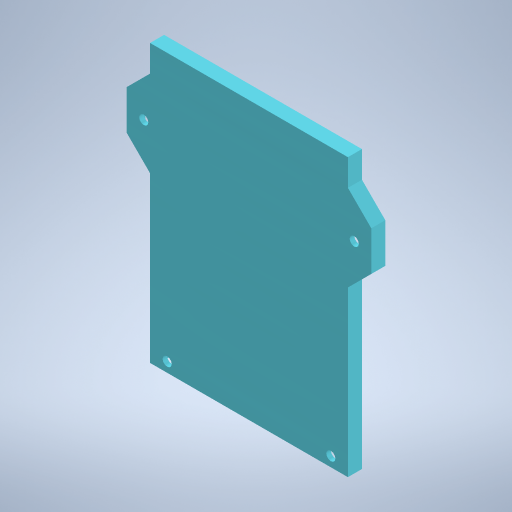
# Autodesk Inventor part: Cover
Saved by Autodesk Inventor 2024.2 (Build 282272000, 272)
## iProperties
Created: 2024-06-02
Part Number: Cover
Material: PBT Plastic
Document SubType Name: Modeling
Designer: simon
Density: 1.31 g/cm^3
Appearance: Cadet Blue
Author: simon
Autodesk Inventor part; units mm, degrees
ref_plane "YZ Plane" through (0, 0, 0) normal (1, 0, 0) x (0, 1, 0)
ref_plane "XZ Plane" through (0, 0, 0) normal (0, 1, 0) x (-1, 0, 0)
ref_plane "XY Plane" through (0, 0, 0) normal (0, 0, 1) x (1, 0, 0)
sketch "Sketch3" plane through (0, 0, 0) normal (0, 0, 1) x (1, 0, 0)
  line L0 (-10, 81) -> (0, 71) projected
  line L1 (-10, 96) -> (-10, 81) projected
  line L2 (0, 106) -> (-10, 96) projected
  line L3 (0, 116) -> (0, 106) projected
  line L4 (80, 116) -> (0, 116) projected
  line L5 (80, 106) -> (80, 116) projected
  line L6 (90, 96) -> (80, 106) projected
  line L7 (90, 81) -> (90, 96) projected
  line L8 (80, 71) -> (90, 81) projected
  line L9 (80, -0.1962) -> (80, 71) projected
  circle A0 centre (85, 88.5) radius 1.95 projected
  circle A1 centre (75, 4) radius 1.95 projected
  circle A2 centre (5, 4) radius 1.95 projected
  circle A3 centre (-5, 88.5) radius 1.95 projected
  line L10 (80, -0.1962) -> (80, 71)
  line L11 (80, 71) -> (90, 81)
  line L12 (90, 81) -> (90, 96)
  line L13 (90, 96) -> (80, 106)
  line L14 (80, 106) -> (80, 116)
  line L15 (80, 116) -> (0, 116)
  line L16 (0, 116) -> (0, 106)
  line L17 (0, 106) -> (-10, 96)
  line L18 (-10, 96) -> (-10, 81)
  line L19 (-10, 81) -> (0, 71)
  line L20 (80, -0.1962) -> (0, -0.1962)
  line L21 (0, 71) -> (0, -0.1962) projected
  line L22 (0, -0.1962) -> (0, 71)
  circle A4 centre (5, 4) radius 1.65
  circle A5 centre (-5, 88.5) radius 1.65
  circle A6 centre (85, 88.5) radius 1.65
  circle A7 centre (75, 4) radius 1.65
  line L23 (0, -0.1962) -> (-2.3, -0.1962)
  line L24 (-2.3, -0.1962) -> (-2.3, 70.0473)
  line L25 (-2.3, 70.0473) -> (-12.3, 80.0473)
  line L26 (-12.3, 80.0473) -> (-12.3, 96.9527)
  line L27 (-12.3, 96.9527) -> (-2.3, 106.9527)
  line L28 (-2.3, 106.9527) -> (-2.3, 118.3)
  line L29 (-2.3, 118.3) -> (82.3, 118.3)
  line L30 (82.3, 118.3) -> (82.3, 106.9527)
  line L31 (82.3, 106.9527) -> (92.3, 96.9527)
  line L32 (92.3, 96.9527) -> (92.3, 80.0473)
  line L33 (92.3, 80.0473) -> (82.3, 70.0473)
  line L34 (82.3, 70.0473) -> (82.3, -0.1962)
  line L35 (82.3, -0.1962) -> (80, -0.1962)
  point P0 (0, 0)
  dimension "d10" = 3.3
  dimension "d11" = 3.3
  dimension "d12" = 3.3
  dimension "d13" = 3.3
  dimension "d14" = 2.3
  dimension "d15" = 2.3
  dimension "d16" = 2.3
  dimension "d17" = 2.3
  dimension "d18" = 2.3
  dimension "d19" = 2.3
  dimension "d20" = 2.3
  dimension "d21" = 2.3
  dimension "d22" = 2.3
  dimension "d23" = 2.3
  dimension "d24" = 2.3
  constraints: 50 end point, 12 parallel, 10 perpendicular, 7 collinear, 4 centre point, 4 coincident, 1 horizontal, 1 point on line, 1 vertical
  measures "d10" diameter of A4
  measures "d11" diameter of A5
  measures "d12" diameter of A6
  measures "d13" diameter of A7
  measures "d14" distance of L20.end L23.end
  measures "d15" distance between parallel lines of L25 L0
  measures "d16" distance between parallel lines of L26 L1
  measures "d17" distance between parallel lines of L27 L2
  measures "d18" distance between parallel lines of L28 L3
  measures "d19" distance between parallel lines of L29 L4
  measures "d20" distance between parallel lines of L30 L5
  measures "d21" distance between parallel lines of L6 L31
  measures "d22" distance between parallel lines of L7 L32
  measures "d23" distance between parallel lines of L33 L11
  measures "d24" distance between parallel lines of L9 L34
extrude "Extrusion2" add sketch "Sketch3" along normal blind 2 contours L1 L2 L3 L4 L5 L6 L7 L8 L9 L20 L21 L0 | L0 L21 L23 L24 L25 L26 L27 L28 L29 L30 L31 L32 L33 L34 L35 L9 L8 L7 L6 L5 L4 L3 L2 L1
sketch "Sketch4" plane through (0, 0, 0) normal (0, 0, -1) x (-1, 0, 0)
  line L0 (2.3, 70.0473) -> (2.3, -0.1962) projected
  line L1 (2.3, -0.1962) -> (0.3, -0.1962)
  line L2 (2.3, -0.1962) -> (-82.3, -0.1962) projected
  line L3 (2.3, -0.1962) -> (2.3, 70.0473)
  line L4 (12.3, 80.0473) -> (2.3, 70.0473) projected
  line L5 (2.3, 70.0473) -> (12.3, 80.0473)
  line L6 (12.3, 96.9527) -> (12.3, 80.0473) projected
  line L7 (12.3, 80.0473) -> (12.3, 96.9527)
  line L8 (12.3, 96.9527) -> (2.3, 106.9527)
  line L9 (2.3, 118.3) -> (2.3, 106.9527) projected
  line L10 (2.3, 106.9527) -> (2.3, 118.3)
  line L11 (2.3, 118.3) -> (-82.3, 118.3)
  line L12 (-82.3, 106.9527) -> (-82.3, 118.3) projected
  line L13 (-82.3, 118.3) -> (-82.3, 106.9527)
  line L14 (-82.3, 106.9527) -> (-92.3, 96.9527)
  line L15 (-82.3, 70.0473) -> (-92.3, 80.0473) projected
  line L16 (-92.3, 96.9527) -> (-92.3, 80.0473)
  line L17 (-92.3, 80.0473) -> (-82.3, 70.0473)
  line L18 (-82.3, 70.0473) -> (-82.3, -0.1962)
  line L19 (-82.3, -0.1962) -> (-80.3, -0.1962)
  line L20 (-80.3, -0.1962) -> (-80.3, 70.8757)
  line L21 (-80.3, 70.8757) -> (-90.3, 80.8757)
  line L22 (-90.3, 80.8757) -> (-90.3, 96.1243)
  line L23 (-90.3, 96.1243) -> (-80.3, 106.1243)
  line L24 (-80.3, 106.1243) -> (-80.3, 116.3)
  line L25 (-80.3, 116.3) -> (0.3, 116.3)
  line L26 (0.3, 116.3) -> (0.3, 106.1243)
  line L27 (0.3, 106.1243) -> (10.3, 96.1243)
  line L28 (10.3, 96.1243) -> (10.3, 80.8757)
  line L29 (10.3, 80.8757) -> (0.3, 70.8757)
  line L30 (0.3, 70.8757) -> (0.3, -0.1962)
  line L31 (2.3, 70.0473) -> (2.3, -0.1962) projected
  line L32 (12.3, 80.0473) -> (2.3, 70.0473) projected
  line L33 (12.3, 96.9527) -> (12.3, 80.0473) projected
  line L34 (2.3, 106.9527) -> (12.3, 96.9527) projected
  line L35 (2.3, 118.3) -> (2.3, 106.9527) projected
  line L36 (-82.3, 118.3) -> (2.3, 118.3) projected
  line L37 (-82.3, 106.9527) -> (-82.3, 118.3) projected
  line L38 (-92.3, 96.9527) -> (-82.3, 106.9527) projected
  line L39 (-92.3, 80.0473) -> (-92.3, 96.9527) projected
  line L40 (-82.3, 70.0473) -> (-92.3, 80.0473) projected
  line L41 (-82.3, -0.1962) -> (-82.3, 70.0473) projected
  line L42 (2.3, 106.9527) -> (12.3, 96.9527)
  line L43 (2.3, 106.9527) -> (12.3, 96.9527)
  line L44 (2.3, 70.0473) -> (12.3, 80.0473)
  line L45 (-82.3, 106.9527) -> (-92.3, 96.9527)
  line L46 (-92.3, 80.0473) -> (-92.3, 96.9527) projected
  line L47 (-82.3, 106.9527) -> (-92.3, 96.9527)
  point P0 (0, 0)
  point P1 (12.3, 88.5)
  dimension "d27" = 2
  dimension "d28" = 2
  dimension "d29" = 2
  dimension "d30" = 2
  dimension "d31" = 2
  dimension "d32" = 2
  dimension "d33" = 2
  dimension "d34" = 2
  dimension "d35" = 2
  dimension "d36" = 2
  constraints: 58 end point, 19 parallel, 9 collinear, 5 perpendicular, 5 point on line, 1 midpoint
  measures "d27" distance of L0.end L1.end
  measures "d28" distance of L2.end L19.end
  measures "d29" distance between parallel lines of L32 L29
  measures "d30" distance from line of point (12.3, 88.5) L28
  measures "d31" distance between parallel lines of L34 L27
  measures "d32" distance between parallel lines of L26 L35
  measures "d33" distance between parallel lines of L36 L25
  measures "d34" distance between parallel lines of L38 L23
  measures "d35" distance between parallel lines of L39 L22
  measures "d36" distance between parallel lines of L40 L21
extrude "Extrusion3" add sketch "Sketch4" along normal blind 4 contours L0 L1 L30 L29 L28 L27 L26 L25 L24 L23 L22 L21 L20 L2 L18 L15 L16 L14 L12 L11 L9 L8 L6 L4
body "Solid2"
